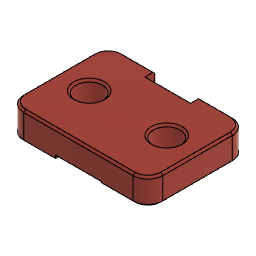
[a]_z_belt_clip_upper_x4 (Autodesk Fusion 360 design; units mm, degrees)
Autodesk Fusion 360 part; units mm, degrees
note: some values were not read from the file. Set by a fixed rule: which sketch regions a step uses.
sketch "Sketch1" plane through (0, 0, 0) normal (0, 0, 1) x (1, 0, 0) in component "[a]_z_belt_clip_upper_x4"
  line L0 (14, -10) -> (-14, -10)
  line L1 (-14, -10) -> (-14, 10)
  line L2 (-14, 10) -> (14, 10)
  line L3 (14, 10) -> (14, -10)
  line L4 (14, -10) -> (-14, 10) construction
  line L5 (-14, -10) -> (14, 10) construction
  circle A0 centre (-7.8, 0) radius 2.7
  circle A1 centre (7.8, 0) radius 2.7
  dimension "d4" = 28
  dimension "d5" = 20
  dimension "d6" = 5.4
  dimension "d7" = 5.4
  dimension "d8" = 6.2
  dimension "d9" = 6.2
  constraint horizontal L0
  constraint perpendicular L0 L1
  constraint parallel L0 L2
  constraint parallel L1 L3
  constraint coincident L4 origin
  constraint coincident L5 origin
  measures "d4" distance of L1.end L2.end
  measures "d5" distance of L0.end L1.end
  measures "d6" diameter of A0
  measures "d7" diameter of A1
  measures "d8" distance of L1 A0.centre
  measures "d9" distance of L3 A1.centre
extrude "Extrude1" add sketch "Sketch1" along normal mid plane 5.2 in component "[a]_z_belt_clip_upper_x4"
fillet "Fillet1" radius 3 4 edges at (14, -10, 0) (14, 10, 0) (-14, -10, 0) (-14, 10, 0) in component "[a]_z_belt_clip_upper_x4"
sketch "Sketch2" plane through (0, 0, 2.6) normal (0, 0, 1) x (-1, 0, 0) in component "[a]_z_belt_clip_upper_x4"
  arc A0 (11, -10) -> (14, -7) centre (11, -7) ccw
  line L0 (14, -7) -> (14, 7)
  arc A1 (14, 7) -> (11, 10) centre (11, 7) ccw
  line L1 (11, 10) -> (-11, 10)
  arc A2 (-11, 10) -> (-14, 7) centre (-11, 7) ccw
  line L2 (-14, 7) -> (-14, -7)
  arc A3 (-14, -7) -> (-11, -10) centre (-11, -7) ccw
  line L3 (-11, -10) -> (11, -10)
  circle A4 centre (-7.8, 0) radius 2.7
  circle A5 centre (7.8, 0) radius 2.7
  line L4 (-4.6, -9) -> (4.6, -9)
  line L5 (4.6, -9) -> (4.6, -10)
  line L6 (4.6, -10) -> (-4.6, -10)
  line L7 (-4.6, -10) -> (-4.6, -9)
  line L8 (-4.6, -9) -> (4.6, -10) construction
  line L9 (4.6, -9) -> (-4.6, -10) construction
  line L10 (0, 0) -> (0, -20) construction
  point P0 (0, -9.5)
  dimension "d14" = 9.2
  dimension "d15" = 1
  constraint horizontal L4
  constraint perpendicular L4 L5
  constraint parallel L4 L6
  constraint parallel L5 L7
  constraint coincident L8 P0
  constraint coincident L9 P0
  constraint coincident L10.start origin
  constraint vertical L10
  constraint coincident P0 L10
  constraint collinear L3 L6
  measures "d14" distance of L5.end L6.end
  measures "d15" distance of L4.end L5.end
extrude "Extrude2" cut sketch "Sketch2" along normal through all and the other way through all contours L3 L4 L5 L6 L7 in component "[a]_z_belt_clip_upper_x4"
sketch "Sketch3" plane through (0, 0, -2.6) normal (0, 0, -1) x (1, 0, 0) in component "[a]_z_belt_clip_upper_x4"
  line L0 (4.6, -9) -> (4.6, -10)
  line L1 (4.6, -10) -> (11, -10)
  arc A0 (11, -10) -> (14, -7) centre (11, -7) ccw
  line L2 (14, -7) -> (14, 7)
  arc A1 (14, 7) -> (11, 10) centre (11, 7) ccw
  line L3 (11, 10) -> (-11, 10)
  arc A2 (-11, 10) -> (-14, 7) centre (-11, 7) ccw
  line L4 (-14, 7) -> (-14, -7)
  arc A3 (-14, -7) -> (-11, -10) centre (-11, -7) ccw
  line L5 (-11, -10) -> (-4.6, -10)
  line L6 (-4.6, -10) -> (-4.6, -9)
  line L7 (-4.6, -9) -> (4.6, -9)
  circle A4 centre (7.8, 0) radius 2.7
  circle A5 centre (-7.8, 0) radius 2.7
  line L8 (7.6, -2) -> (-7.6, -2)
  line L9 (-7.6, -2) -> (-7.6, 2)
  line L10 (-7.6, 2) -> (7.6, 2)
  line L11 (7.6, 2) -> (7.6, -2)
  line L12 (7.6, -2) -> (-7.6, 2) construction
  line L13 (-7.6, -2) -> (7.6, 2) construction
  line L14 (4.6, -10) -> (-4.6, -10)
  line L15 (-4.6, -10) -> (-4.6, 10)
  line L16 (-4.6, 10) -> (4.6, 10)
  line L17 (4.6, 10) -> (4.6, -10)
  line L18 (4.6, -10) -> (-4.6, 10) construction
  line L19 (-4.6, -10) -> (4.6, 10) construction
  dimension "d17" = 4
  dimension "d18" = 15.2
  constraint horizontal L8
  constraint perpendicular L8 L9
  constraint parallel L8 L10
  constraint parallel L9 L11
  constraint coincident L12 origin
  constraint coincident L13 origin
  constraint horizontal L14
  constraint perpendicular L14 L15
  constraint parallel L14 L16
  constraint parallel L15 L17
  constraint coincident L0.end L1.start
  constraint coincident L18 origin
  constraint coincident L19 origin
  measures "d17" distance of L8.end L9.end
  measures "d18" distance of L9.end L10.end
extrude "Extrude3" cut sketch "Sketch3" against normal blind 0.6 contours L0 L6 L7 L14 L15 L17 | L7 L8 L15 L17 | A4 L8 L10 L17 | L8 L10 L15 L17 | A5 L8 L10 L15 | A4 L8 L10 L11 | L3 L10 L15 L16 L17 | A5 L8 L9 L10 picked at (8.5667, 0) picked at (-6.7667, 0) in component "[a]_z_belt_clip_upper_x4"
chamfer "Chamfer1" distance 0.4 angle 45 16 edges at (-10.3173, 0.9764, 2.6) (5.2827, 0.9764, 2.6) (14, 0, 2.6) (13.1213, -9.1213, 2.6) (0, -10, 2.6) (-13.1213, -9.1213, 2.6) (-14, 0, 2.6) (-13.1213, 9.1213, 2.6) (-7.8, 10, 2.6) (7.8, 10, 2.6) (13.1213, 9.1213, 2.6) (7.8, -10, -2.6) (7.8, 10, -2.6) (13.1213, 9.1213, -2.6) (14, 0, -2.6) (13.1213, -9.1213, -2.6) in component "[a]_z_belt_clip_upper_x4"
chamfer "Chamfer2" distance 1 angle 45 2 edges at (0, 9, 2.6) (0, 9, -2) in component "[a]_z_belt_clip_upper_x4"
component "[a]_z_belt_clip_upper_x4" placed x (1, 0, 0) y (0, 1, 0) z (0, 0, 1) at (0, 0, 0)
equation "tolerance = 0.2 mm"
equation "chamfer = 0.4 mm"
equation "z_belt_width = 9 mm"
equation "d4 = z_belt_width + 19 mm"
equation "d10 = ( 5.2 / 2 ) * 1 mm"
equation "d14 = z_belt_width + tolerance"
equation "d18 = z_belt_width + tolerance + 6 mm"
equation "d21 = chamfer"
